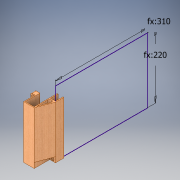
# Autodesk Inventor part: AufnahmeLinks
Saved by Autodesk Inventor 2019 (Build 230136000, 136)
## iProperties
Created: 2019-03-02
Part Number: AufnahmeLinks
Material: Generisch
Document SubType Name: Modeling
Designer: Thomas
Density: 1 g/cm^3
Appearance: Kirsche - natur - schwacher Glanz
Author: Thomas
Autodesk Inventor part; units mm, degrees
ref_plane "YZ Plane" through (0, 0, 0) normal (1, 0, 0) x (0, 1, 0)
ref_plane "XZ Plane" through (0, 0, 0) normal (0, 1, 0) x (-1, 0, 0)
ref_plane "XY Plane" through (0, 0, 0) normal (0, 0, 1) x (1, 0, 0)
sketch "Skizze1" plane through (0, 0, 0) normal (0, 0, 1) x (1, 0, 0)
  line L0 (-26.25, -95) -> (26.25, -95)
  line L1 (26.25, -95) -> (26.25, 95)
  line L2 (26.25, 95) -> (-26.25, 95)
  line L3 (-26.25, 95) -> (-26.25, -95)
  line L4 (-38.4, 0) -> (46.65, 0) projected
  line L5 (0, -140.5) -> (0, 178) projected
  dimension "d0" = 52.5
  dimension "d1" = 190
  constraints: 8 end point, 2 parallel, 1 horizontal, 1 perpendicular, 2 other
  measures "d0" distance of L1.end L2.end
  measures "d1" distance of L2.end L0.start
sketch "Skizze2" plane through (0, 0, 0) normal (0, 1, 0) x (-1, 0, 0)
  line L0 (39, 0) -> (-50.25, 0) projected
  line L1 (0, -228.1) -> (0, 283.6) projected
  line L2 (18, 158) -> (18, 210.5)
  line L3 (18, 210.5) -> (-18, 210.5)
  line L4 (-18, 210.5) -> (-18, 158)
  line L5 (-18, 158) -> (-37.5, 158)
  line L6 (-37.5, 158) -> (-37.5, 130)
  line L7 (-37.5, 130) -> (-34.5, 130)
  line L8 (-34.5, 130) -> (-34.5, 155)
  line L9 (-34.5, 155) -> (-15, 155)
  line L10 (-15, 155) -> (-15, 207.5)
  line L11 (-15, 207.5) -> (15, 207.5)
  line L12 (15, 207.5) -> (15, 158)
  line L13 (15, 158) -> (18, 158)
  line L14 (-15, 155) -> (-18, 155)
  line L15 (-18, 155) -> (-18, 130)
  line L16 (-18, 130) -> (-15, 130)
  line L17 (-15, 130) -> (-15, 155)
  point P0 (0, 0)
  dimension "d2" = 3
  dimension "d3" = 3
  dimension "d4" = 3
  dimension "d5" = 3
  dimension "d6" = 3
  dimension "d7" = 30
  dimension "d8" = 19.5
  dimension "d9" = 77.5
  dimension "d10" = 25
  dimension "d11" = 207.5
  constraints: 33 end point, 11 perpendicular, 2 collinear, 2 parallel, 2 point on line, 1 horizontal, 1 vertical, 1 other
  measures "d2" distance between parallel lines of L2 L12
  measures "d3" distance between parallel lines of L3 L11
  measures "d4" distance between parallel lines of L4 L10
  measures "d5" distance between parallel lines of L9 L5
  measures "d6" distance between parallel lines of L6 L8
  measures "d7" distance of L10.end L11.end
  measures "d8" distance of L8.end L9.end
  measures "d9" distance between parallel lines of L7 L11
  measures "d10" distance between parallel lines of L7 L9
  measures "d11" distance between parallel lines of L0 L11
extrude "Extrusion1" add sketch "Skizze2" along normal mid plane 175
sketch "Skizze3" plane through (0, -87.5, 0) normal (0, -1, 0) x (1, 0, 0)
  line L0 (-18, 210.5) -> (-18, 158) projected
  line L1 (-18, 158) -> (-15, 158) projected
  line L2 (-15, 158) -> (-15, 207.5) projected
  line L3 (-15, 207.5) -> (15, 207.5) projected
  line L4 (15, 207.5) -> (15, 130) projected
  line L5 (18, 155) -> (34.5, 155) projected
  line L6 (34.5, 155) -> (34.5, 130) projected
  line L7 (34.5, 130) -> (37.5, 130) projected
  line L8 (37.5, 130) -> (37.5, 158) projected
  line L9 (37.5, 158) -> (18, 158) projected
  line L10 (18, 158) -> (18, 210.5) projected
  line L11 (18, 210.5) -> (-18, 210.5) projected
  line L12 (34.5, 130) -> (34.5, 155) projected
  line L13 (34.5, 155) -> (15, 155)
  line L14 (15, 155) -> (15, 130)
  line L15 (15, 130) -> (34.5, 130)
  line L16 (34.5, 130) -> (34.5, 155)
  line L17 (15, 130) -> (18, 130) projected
  line L18 (18, 130) -> (18, 155) projected
  line L19 (15, 130) -> (15, 207.5) projected
  constraints: 8 end point, 2 parallel, 1 collinear, 1 horizontal, 1 perpendicular
extrude "Extrusion2" add sketch "Skizze3" along normal blind 3
sketch "Skizze8" plane through (0, -87.5, 0) normal (0, 1, 0) x (1, 0, 0)
  line L0 (18, -130) -> (18, -155) projected
  line L1 (18, -155) -> (34.5, -155) projected
  line L2 (34.5, -155) -> (34.5, -130) projected
  line L3 (18, -130) -> (34.5, -130) projected
extrude "Extrusion5" add sketch "Skizze8" along normal blind 11
sketch "Skizze9" plane through (18, 87.5, 158) normal (0, 0, 1) x (1, 0, 0)
  circle A0 centre (9.75, -171) radius 3.75
  line L0 (19.5, 0) -> (19.5, -178) construction
  line L1 (0, 0) -> (19.5, 0) projected
  line L2 (0, 0) -> (0, -178) construction
  line L3 (19.5, -178) -> (0, -178) construction
  line L4 (16.5, -164) -> (0, -164) construction
  line L5 (0, -164) -> (19.5, -164) construction
  line L6 (19.5, -164) -> (19.5, -178) construction
  line L7 (19.5, -178) -> (0, -178) construction
  line L8 (0, -178) -> (0, -164) construction
  line L9 (0, 0) -> (0, -178) projected
  line L10 (0, -178) -> (19.5, -164) construction
  line L11 (0, -164) -> (19.5, -178) construction
  dimension "d34" = 7.5
  constraints: 12 end point, 2 collinear, 2 point on line, 1 centre point, 1 coincident, 1 midpoint, 1 perpendicular
  measures "d34" diameter of A0
extrude "Extrusion6" cut sketch "Skizze9" against normal through all
chamfer "Fase1" distance 1 angle 45 2 edges at (24, -83.5, 158) (24, -83.5, 130)
sketch "Skizze10" plane through (-18, 87.5, 158) normal (-1, 0, 0) x (0, 0, 1)
  line L0 (0, 0) -> (52.5, 0) projected
  line L1 (52.5, -178) -> (52.5, 0) projected
  line L2 (0, 0) -> (52.5, 0) projected
  line L3 (0, 0) -> (0, -178) projected
  line L4 (52.5, -178) -> (0, -178) projected
  line L5 (0, 0) -> (14, 0)
  line L6 (14, 0) -> (14, -14)
  line L7 (14, -14) -> (0, -14)
  line L8 (0, -14) -> (0, 0)
  dimension "d40" = 14
  dimension "d41" = 14
  constraints: 8 end point, 2 parallel, 1 horizontal, 1 perpendicular
  measures "d40" distance of L6.end L7.end
  measures "d41" distance of L5.end L6.end
extrude "Extrusion7" add sketch "Skizze10" along normal blind 14 contours L0 L6 L7 L3
fillet "Rundung2" radius 16 1 edges at (-18, 73.5, 165)
fillet "Rundung2" radius 4 1 edges at (-32, 73.5, 165)
fillet "Rundung2" radius 4 1 edges at (-32, 87.5, 165)
sketch "Skizze11" plane through (-32, 87.5, 172) normal (0, 0, 1) x (1, 0, 0)
  circle A0 centre (7, -7) radius 7
  arc A1 (0, -10.7957) -> (2.8, -14.6115) centre (4, -10.7957) ccw projected
  arc A2 (14, -29.8745) -> (2.8, -14.6115) centre (-2, -29.8745) ccw projected
  line L0 (14, 0) -> (14, -29.8745) projected
  line L1 (14, 0) -> (4, 0) projected
  line L2 (0, -10.7957) -> (0, -4) projected
  line L3 (14, 0) -> (4, 0) projected
  line L4 (0, -10.7957) -> (0, -4) projected
  circle A3 centre (7, -7) radius 3.75
  arc A4 (4, 0) -> (0, -4) centre (4, -4) ccw projected
  point P0 (0, 0)
  dimension "d46" = 7
  dimension "d47" = 7.5
  constraints: 2 centre point, 2 tangent, 1 coincident
  measures "d46" distance from line of A0.centre L1
  measures "d47" diameter of A3
extrude "Extrusion8" cut sketch "Skizze11" against normal through all contours A3
sketch "Skizze4" plane through (34.5, 87.5, 130) normal (-1, 0, 0) x (0, 0, 1)
  line L0 (25, 0) -> (25, -175) projected
  line L1 (25, -175) -> (-285, -175)
  line L2 (-285, -175) -> (-285, 45)
  line L3 (-285, 45) -> (25, 45)
  line L4 (25, 45) -> (25, -175)
  dimension "d16" = 310
  dimension "d17" = 220
  constraints: 8 end point, 2 parallel, 1 horizontal, 1 perpendicular
  measures "d16" distance of L2.end L3.end
  measures "d17" distance of L1.end L2.end
sketch "Skizze5" plane through (-18, 87.5, 158) normal (-1, 0, 0) x (0, 0, 1)
  line L0 (6, -5) -> (46.5, -5) construction
  line L1 (6, -2.75) -> (46.5, -2.75)
  line L2 (46.5, -7.25) -> (6, -7.25)
  arc A0 (6, -2.75) -> (6, -7.25) centre (6, -5) ccw
  arc A1 (46.5, -7.25) -> (46.5, -2.75) centre (46.5, -5) ccw
  line L3 (-313, 45) -> (-3, 45) projected
  line L4 (0, 0) -> (0, -178) projected
  line L5 (52.5, -178) -> (52.5, 0) projected
  point P0 (26.25, -5)
  dimension "d18" = 4.5
  dimension "d19" = 50
  dimension "d20" = 6
  dimension "d21" = 6
  constraints: 8 end point, 4 point on circle, 4 tangent, 2 centre point, 1 horizontal, 1 midpoint, 1 parallel
  measures "d18" distance between parallel lines of L1 L2
  measures "d19" distance between parallel lines of L0 L3
  measures "d20" distance from line of L4 L0.start
  measures "d21" distance from line of L5 L0.end
extrude "Extrusion3" [suppressed]
pattern_linear "Rechteckige Anordnung1" [suppressed]
sketch "Skizze13" plane through (0, 87.5, 0) normal (0, 1, 0) x (1, 0, 0)
  line L0 (37.5, -158) -> (37.5, -130) projected
  line L1 (37.5, -158) -> (18, -210.5)
  line L2 (18, -210.5) -> (15.1877, -209.4554)
  line L3 (15.1877, -209.4554) -> (34.6877, -156.9554)
  line L4 (34.6877, -156.9554) -> (37.5, -158)
  line L5 (18, -210.5) -> (18, -158) projected
  line L6 (15, -130) -> (15, -207.5) projected
  dimension "d51" = 3
  dimension "d52" = 3
  constraints: 8 end point, 2 parallel, 1 perpendicular
  measures "d51" distance between parallel lines of L5 L6
  measures "d52" distance between parallel lines of L1 L3
extrude "Extrusion9" add sketch "Skizze13" against normal blind 160
fillet "Rundung3" radius 7 2 edges at (34.2997, 7.5, 158) (18, -1.5, 158)
sketch "Skizze14" plane through (0, -90.5, 0) normal (0, -1, 0) x (1, 0, 0)
  line L0 (18, 201.8839) -> (18, 165) projected
  line L1 (37.5013, 157.9968) -> (18, 157.9968)
  line L2 (18, 157.9968) -> (18, 175.3621)
  line L3 (18, 175.3621) -> (37.5013, 175.3621)
  line L4 (37.5013, 175.3621) -> (37.5013, 157.9968)
  constraints: 8 end point, 2 parallel, 1 horizontal, 1 perpendicular, 1 point on line
extrude "Extrusion10" cut sketch "Skizze14" against normal up to surface (18 mm away)
equation "\"d0\" = -0.5 * BreiteTablet + 0.5 * BreitePanel"
equation "\"d2\" = Materialstaerke"
equation "\"d3\" = d2"
equation "\"d4\" = d3"
equation "\"d5\" = d2"
equation "\"d6\" = d5"
equation "\"d7\" = DickePanel"
equation "\"d8\" = DickeTablet + Materialstaerke"
equation "\"d9\" = 0.5 * BreitePanel - 0.5 * BreiteTablet + BreiteRahmenTabletScreen"
equation "\"d10\" = BreiteRahmenTabletScreen"
equation "\"d11\" = 0.5 * BreitePanel"
equation "\"d14\" = Materialstaerke"
equation "\"d41\" = d40"
equation "\"d16\" = BreiteTablet"
equation "\"d17\" = HöheTablet"
equation "\"d18\" = DurchmesserLoch"
equation "\"d19\" = VersatzSchraubeOberkanteTB"
equation "\"d20\" = 2 * Materialstaerke"
equation "\"d21\" = 2 * Materialstaerke"
equation "\"d22\" = Materialstaerke"
equation "\"d26\" = AbstandLochbild"
equation "\"d52\" = d51"
equation "\"BreiteTablet\" = 310"
equation "\"HöheTablet\" = 220"
equation "\"DickeTablet\" = 16.5"
equation "\"BreitePanel\" = 415"
equation "\"DickePanel\" = 30"
equation "\"AbstandLochbild\" = 150"
equation "\"DurchmesserLoch\" = 4.5"
equation "\"VersatzSchraubeOberkanteTB\" = 50"
equation "\"Materialstaerke\" = 3"
equation "\"BreiteRahmenTabletScreen\" = 25"
